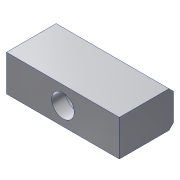
# Autodesk Inventor part: Jaw
Saved by Autodesk Inventor 2016 (Build 200138000, 138)
## iProperties
Created: 2015-08-18
Part Number: Jaw
Material: Aluminum 6061
Document SubType Name: Modeling
Density: 2.7 g/cm^3
Appearance: Aluminum - Flat
Autodesk Inventor part; units mm, degrees
ref_plane "YZ Plane" through (0, 0, 0) normal (1, 0, 0) x (0, 1, 0)
ref_plane "XZ Plane" through (0, 0, 0) normal (0, 1, 0) x (-1, 0, 0)
ref_plane "XY Plane" through (0, 0, 0) normal (0, 0, 1) x (1, 0, 0)
sketch "Sketch1" plane through (0, 0, 0) normal (1, 0, 0) x (0, 1, 0)
  line L0 (-6, -4) -> (6, -4)
  line L1 (6, -4) -> (6, 4)
  line L2 (6, 4) -> (-6, 4)
  line L3 (-6, 4) -> (-6, -4)
  line L4 (-6, -4) -> (6, 4) construction
  line L5 (6, -4) -> (-6, 4) construction
  point P0 (0, 0)
  dimension "d0" = 12
  dimension "d1" = 8
  constraints: 12 end point, 2 midpoint, 2 parallel, 1 horizontal, 1 perpendicular
  measures "d0" distance of L2.end L1.end
  measures "d1" distance of L1.end L0.end
extrude "Extrusion1" add sketch "Sketch1" along normal blind 25
sketch "Sketch2" plane through (0, -6, -4) normal (0, -1, 0) x (1, 0, 0)
  line L0 (0, 8) -> (25, 8) projected
  line L1 (0, 8) -> (0, 0) projected
  point P0 (0, 4)
  point P1 (12.5, 4)
  point P2 (12.5, 8)
  point P3 (0, 4)
  constraints: 2 midpoint, 1 horizontal alignment, 1 vertical alignment
hole "Hole1" at (12.5, -6, 0) direction (0, 1, 0) diameter 5 depth 3 tip angle 118
chamfer "Chamfer1" distance 1 angle 45 2 edges at (12.5, 6, -4) (12.5, 6, 4)
body "Solid1"
